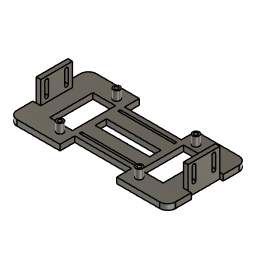
Plataforma_teorica_control_prueba v17 (Autodesk Fusion 360 design; units mm, degrees)
Autodesk Fusion 360 part; units mm, degrees
note: some values were not read from the file. Set by a fixed rule: which sketch regions a step uses.
sketch "Boceto1" plane through (0, 0, 0) normal (0, 0, 1) x (1, 0, 0)
  line L0 (0, 0) -> (80, 0) construction
  line L1 (80, 0) -> (80, 60) construction
  line L2 (80, 60) -> (0, 60) construction
  line L3 (0, 60) -> (0, 0) construction
  circle A0 centre (5, 55) radius 1.625
  circle A1 centre (75, 55) radius 1.625
  line L4 (110, -5) -> (-30, -5)
  line L5 (-30, -5) -> (-30, 65)
  line L6 (-30, 65) -> (110, 65)
  line L7 (110, 65) -> (110, -5)
  line L8 (15, 46) -> (65, 46)
  line L9 (65, 46) -> (65, 48)
  line L10 (65, 48) -> (15, 48)
  line L11 (15, 48) -> (15, 46)
  line L12 (-30, 30) -> (115, 30)
  line L13 (110, 30) -> (107, 30)
  line L14 (107, 30) -> (107, 44)
  line L15 (107, 44) -> (110, 44)
  line L16 (110, 44) -> (110, 30)
  line L17 (110, 16) -> (110, 30)
  line L18 (110, 30) -> (107, 30)
  line L19 (107, 16) -> (110, 16)
  line L20 (107, 30) -> (107, 16)
  line L21 (40, 65) -> (40, -5)
  circle A2 centre (5, 5) radius 1.625
  circle A3 centre (75, 5) radius 1.625
  line L22 (-30, 44) -> (-30, 30)
  line L23 (-30, 30) -> (-27, 30)
  line L24 (-27, 30) -> (-27, 44)
  line L25 (-27, 44) -> (-30, 44)
  line L26 (-30, 16) -> (-30, 30)
  line L27 (-30, 30) -> (-27, 30)
  line L28 (-27, 16) -> (-30, 16)
  line L29 (-27, 30) -> (-27, 16)
  line L30 (65, 12) -> (15, 12)
  line L31 (15, 12) -> (15, 14)
  line L32 (15, 14) -> (65, 14)
  line L33 (65, 14) -> (65, 12)
  dimension "d1" = 80
  dimension "d2" = 60
  dimension "d3" = 5
  dimension "d4" = 70
  dimension "d8" = 3.25
  dimension "d16" = 70
  dimension "d17" = 140
  dimension "d19" = 30
  dimension "d20" = 5
  dimension "d29" = 7
  dimension "d31" = 2
  dimension "d34" = 50
  dimension "d37" = 14
  dimension "d38" = 3
  dimension "d39" = 5
  constraint horizontal L0
  constraint vertical L1
  constraint horizontal L2
  constraint vertical L3
  constraint coincident L0.start L3.end
  constraint horizontal A0.centre A1.centre
  constraint equal A0 A1
  constraint horizontal L4
  constraint vertical L5
  constraint horizontal L6
  constraint vertical L7
  constraint horizontal L8
  constraint vertical L9
  constraint horizontal L10
  constraint vertical L11
  constraint midpoint L5 L12.start
  constraint horizontal L13
  constraint vertical L14
  constraint horizontal L15
  constraint vertical L16
  constraint midpoint L7 L13.start
  constraint symmetric L12 L13.start L16.end
  constraint symmetric L12 L13.end L14.start
  constraint symmetric L12 L14.end L19.start
  constraint symmetric L12 L15.end L17.start
  constraint perpendicular L5 L12
  constraint midpoint L6 L21.start
  constraint perpendicular L0 L21
  constraint midpoint L4 L21.end
  constraint symmetric A0 L12 A2
  constraint symmetric A1 L12 A3
  constraint symmetric L13.start L21 L12.start
  constraint symmetric L13.end L21 L23.end
  constraint symmetric L14.end L21 L24.end
  constraint symmetric L15.end L21 L22.start
  constraint symmetric L17.start L21 L26.start
  constraint symmetric L19.start L21 L28.start
  constraint symmetric L8.start L12 L31.end
  constraint symmetric L8.end L12 L32.end
  constraint symmetric L9.end L12 L30.start
  constraint symmetric L10.end L12 L30.end
  measures "d1" distance of L1.end L2.end
  measures "d2" distance of L0.end L1.end
  measures "d3" horizontal distance of L2.end A0.centre
  measures "d4" distance of A0.centre A1.centre
  measures "d8" diameter of A1
  measures "d16" distance of L4.start L6.end
  measures "d17" distance of L5.end L6.end
  measures "d19" horizontal distance of L0.end L4.start
  measures "d20" vertical distance of L0.end L4.start
  measures "d29" vertical distance of A0.centre L10.end
  measures "d31" distance of L8.end L9.end
  measures "d34" distance of L9.end L10.end
  measures "d37" distance of L13.start L15.end
  measures "d38" distance of L14.end L15.end
  measures "d39" vertical distance of L1.end A1.centre
extrude "Extruir1" add sketch "Boceto1" along normal blind 5 contours L4 L7 L12 L19 L20 L21 L30 L32 L33 | L4 L5 L12 L21 L28 L29 L30 L31 L32 | L6 L7 L8 L9 L10 L12 L14 L15 L21 | L5 L6 L8 L10 L11 L12 L21 L24 L25
sketch "Boceto4" plane through (0, 0, 5) normal (0, 0, 1) x (-1, 0, 0)
  line L0 (-15, -14) -> (-65, -14)
  line L1 (-65, -14) -> (-65, -12)
  line L2 (-65, -12) -> (-15, -12)
  line L3 (-15, -12) -> (-15, -14)
  circle A0 centre (-5, -5) radius 1.625
  circle A1 centre (-75, -55) radius 1.625
  circle A2 centre (-75, -5) radius 1.625
  circle A3 centre (-5, -55) radius 1.625
  line L4 (-15, -46) -> (-15, -48)
  line L5 (-15, -48) -> (-65, -48)
  line L6 (-65, -48) -> (-65, -46)
  line L7 (-65, -46) -> (-15, -46)
  line L8 (27, -44) -> (27, -16)
  line L9 (27, -16) -> (30, -16)
  line L10 (30, -16) -> (30, 5)
  line L11 (30, 5) -> (-110, 5)
  line L12 (-110, 5) -> (-110, -16)
  line L13 (-110, -16) -> (-107, -16)
  line L14 (-107, -16) -> (-107, -44)
  line L15 (-107, -44) -> (-110, -44)
  line L16 (-110, -44) -> (-110, -65)
  line L17 (-110, -65) -> (30, -65)
  line L18 (30, -65) -> (30, -44)
  line L19 (30, -44) -> (27, -44)
  line L20 (-107, -44) -> (-103, -44)
  line L21 (-103, -44) -> (-103, -16)
  line L22 (-103, -16) -> (-107, -16)
  line L23 (-107, -16) -> (-107, -44)
  line L24 (-40, -65) -> (-40, 5)
  line L25 (27, -30) -> (-107, -30)
  line L26 (27, -16) -> (27, -44)
  line L27 (27, -44) -> (23, -44)
  line L28 (23, -44) -> (23, -16)
  line L29 (23, -16) -> (27, -16)
  circle A4 centre (-5, -55) radius 3
  circle A5 centre (-75, -55) radius 3
  circle A6 centre (-5, -5) radius 3
  circle A7 centre (-75, -5) radius 3
  dimension "d42" = 4
  dimension "d58" = 6
  constraint horizontal L20
  constraint vertical L21
  constraint horizontal L22
  constraint vertical L23
  constraint coincident L14.end L15.start
  constraint midpoint L17 L24.start
  constraint midpoint L11 L24.end
  constraint midpoint L8 L25.start
  constraint coincident L13.end L14.start
  constraint symmetric L14.end L24 L8.start
  constraint symmetric L20.end L24 L27.end
  constraint symmetric L21.end L24 L28.end
  constraint symmetric L13.end L24 L8.end
  constraint horizontal L25
  constraint midpoint L23 L25.end
  constraint concentric A3 A4
  constraint symmetric L24 A4 A5
  constraint symmetric L25 A4 A6
  constraint symmetric L25 A5 A7
  measures "d42" distance of L14.end L20.end
  measures "d58" diameter of A4
extrude "Extruir3" add sketch "Boceto4" along normal blind 20 contours L8 L25 L26 L28 L29 | L8 L25 L26 L27 L28 | L14 L21 L22 L23 L25 | L14 L20 L21 L23 L25
extrude "Extruir2" add sketch "Boceto4" along normal blind 10 contours L8 L25 L26 L28 L29 | L8 L25 L26 L27 L28 | L14 L21 L22 L23 L25 | L14 L20 L21 L23 L25
sketch "Boceto5" plane through (107, 0, 0) normal (1, 0, 0) x (0, 1, 0)
  line L0 (16, 0) -> (44, 0)
  line L1 (44, 0) -> (44, 5)
  line L2 (44, 5) -> (44, 25)
  line L3 (16, 25) -> (16, 5)
  line L4 (16, 5) -> (16, 0)
  line L5 (30, 25) -> (30, 0)
  line L6 (44, 25) -> (16, 25)
  line L7 (19.65, 21.5) -> (19.65, 9.5)
  arc A0 (19.65, 9.5) -> (22.85, 9.5) centre (21.25, 9.5) ccw
  line L8 (22.85, 9.5) -> (22.85, 21.5)
  arc A1 (22.85, 21.5) -> (19.65, 21.5) centre (21.25, 21.5) ccw
  line L9 (21.25, 21.5) -> (21.25, 9.5) construction
  arc A2 (37.15, 9.5) -> (40.35, 9.5) centre (38.75, 9.5) ccw
  line L10 (37.15, 9.5) -> (37.15, 21.5)
  arc A3 (40.35, 21.5) -> (37.15, 21.5) centre (38.75, 21.5) ccw
  line L11 (40.35, 21.5) -> (40.35, 9.5)
  dimension "d52" = 3.2
  dimension "d53" = 12
  dimension "d54" = 8.75
  dimension "d55" = 3.5
  constraint midpoint L5.start L6
  constraint midpoint L0 L5.end
  constraint tangent L7 A0
  constraint tangent A0 L8
  constraint parallel L7 L8
  constraint tangent L8 A1
  constraint tangent L7 A1
  constraint vertical L9
  constraint symmetric L5 L7.start A3.start
  constraint symmetric L5 L7.end A2.end
  constraint symmetric L5 A0.end A2.start
  constraint symmetric L5 L8.end L10.end
  constraint symmetric L5 A0 A2
  constraint symmetric L5 A1 A3
  measures "d52" diameter of A0
  measures "d53" distance of A1.centre A0.centre
  measures "d54" horizontal distance of L5.start A1.centre
  measures "d55" vertical distance of L5.start A1.centre
sketch "Boceto2" plane through (0, 0, 0) normal (0, 0, 1) x (1, 0, 0)
sketch "Boceto3" plane through (0, 0, 0) normal (0, 0, 1) x (1, 0, 0)
  point P0 (5, 55)
extrude "Extruir4" cut sketch "Boceto5" against normal blind 155 contours L7 A0 L8 A1 | A2 L10 A3 L11
extrude "Extruir5" add sketch "Boceto4" along normal blind 8 contours A4 | A5 | A6 | A7
sketch "Boceto6" plane through (0, 0, 5) normal (0, 0, 1) x (-1, 0, 0)
  line L0 (10, -30) -> (-10, -30)
  line L1 (-10, -30) -> (-10, -49)
  line L2 (-10, -49) -> (10, -49)
  line L3 (10, -49) -> (10, -30)
  line L4 (-15, -65) -> (-40, -65)
  line L5 (-40, -65) -> (-40, -52)
  line L6 (-40, -52) -> (-15, -52)
  line L7 (-15, -52) -> (-15, -65)
  line L8 (-40, -65) -> (-40, 5)
  line L9 (-90, -49) -> (-90, -30)
  line L10 (-90, -30) -> (-70, -30)
  line L11 (-70, -30) -> (-70, -49)
  line L12 (-70, -49) -> (-90, -49)
  line L13 (27, -30) -> (-107, -30)
  line L14 (-10, -30) -> (-10, -11)
  line L15 (-10, -11) -> (10, -11)
  line L16 (10, -11) -> (10, -30)
  line L17 (10, -30) -> (-10, -30)
  line L18 (-70, -30) -> (-70, -11)
  line L19 (-70, -11) -> (-90, -11)
  line L20 (-90, -11) -> (-90, -30)
  line L21 (-90, -30) -> (-70, -30)
  line L22 (-65, -65) -> (-40, -65)
  line L23 (-40, -65) -> (-40, -52)
  line L24 (-40, -52) -> (-65, -52)
  line L25 (-65, -52) -> (-65, -65)
  line L26 (-15, 5) -> (-40, 5)
  line L27 (-40, 5) -> (-40, -8)
  line L28 (-40, -8) -> (-15, -8)
  line L29 (-15, -8) -> (-15, 5)
  line L30 (-40, -8) -> (-65, -8)
  line L31 (-65, -8) -> (-65, 5)
  line L32 (-65, 5) -> (-40, 5)
  line L33 (-40, 5) -> (-40, -8)
  line L34 (-40, -30) -> (-16, -30)
  line L35 (-16, -30) -> (-16, -35)
  line L36 (-16, -35) -> (-40, -35)
  line L37 (-40, -35) -> (-40, -30)
  line L38 (-40, -30) -> (-64, -30)
  line L39 (-64, -30) -> (-64, -35)
  line L40 (-40, -35) -> (-40, -30)
  line L41 (-64, -35) -> (-40, -35)
  line L42 (-40, -30) -> (-16, -30)
  line L43 (-16, -30) -> (-16, -25)
  line L44 (-16, -25) -> (-40, -25)
  line L45 (-40, -25) -> (-40, -30)
  line L46 (-40, -30) -> (-64, -30)
  line L47 (-64, -30) -> (-64, -25)
  line L48 (-64, -25) -> (-40, -25)
  line L49 (-40, -25) -> (-40, -30)
  arc A0 (-103, 5) -> (-110, -2) centre (-103, -2) ccw
  line L50 (-103, 5) -> (-110, 5)
  line L51 (-110, 5) -> (-110, -2)
  line L52 (30, 5) -> (30, -2)
  line L53 (23, 5) -> (30, 5)
  arc A1 (30, -2) -> (23, 5) centre (23, -2) ccw
  line L54 (-110, -65) -> (-110, -58)
  line L55 (-103, -65) -> (-110, -65)
  arc A2 (-110, -58) -> (-103, -65) centre (-103, -58) ccw
  line L56 (30, -65) -> (30, -58)
  arc A3 (23, -65) -> (30, -58) centre (23, -58) ccw
  line L57 (23, -65) -> (30, -65)
  point P0 (-5, -55)
  point P1 (-75, -5)
  point P2 (-110, 5)
  dimension "d61" = 15
  dimension "d62" = 6
  dimension "d63" = 19
  dimension "d64" = 20
  dimension "d65" = 25
  dimension "d66" = 13
  dimension "d67" = 24
  dimension "d68" = 5
  dimension "d72" = 7
  dimension "d73" = 3
  constraint horizontal L0
  constraint vertical L1
  constraint horizontal L2
  constraint vertical L3
  constraint horizontal L4
  constraint vertical L5
  constraint horizontal L6
  constraint vertical L7
  constraint symmetric L0.start L8 L9.end
  constraint symmetric L0.end L8 L10.end
  constraint symmetric L1.end L8 L11.end
  constraint symmetric L2.end L8 L9.start
  constraint symmetric L0.start L13 L3.end
  constraint symmetric L0.end L13 L1.start
  constraint symmetric L1.end L13 L14.end
  constraint symmetric L2.end L13 L15.end
  constraint symmetric L9.start L13 L19.end
  constraint symmetric L9.end L13 L10.start
  constraint symmetric L10.end L13 L11.start
  constraint symmetric L11.end L13 L18.end
  constraint coincident L4.end L5.start
  constraint symmetric L4.start L8 L22.start
  constraint symmetric L4.end L8 L5.start
  constraint symmetric L5.end L8 L6.start
  constraint symmetric L6.end L8 L24.end
  constraint symmetric L4.start L13 L26.start
  constraint symmetric L4.end L13 L8.end
  constraint symmetric L5.end L13 L27.end
  constraint symmetric L6.end L13 L28.end
  constraint symmetric L13 L22.start L31.end
  constraint symmetric L13 L4.end L8.end
  constraint symmetric L13 L5.end L27.end
  constraint symmetric L13 L24.end L30.end
  constraint horizontal L34
  constraint vertical L35
  constraint horizontal L36
  constraint vertical L37
  constraint midpoint L13 L34.start
  constraint symmetric L8 L34.start L37.end
  constraint symmetric L8 L34.end L38.end
  constraint symmetric L8 L35.end L39.end
  constraint symmetric L8 L36.end L37.start
  constraint symmetric L13 L34.start L37.end
  constraint symmetric L13 L34.end L35.start
  constraint symmetric L13 L35.end L43.end
  constraint symmetric L13 L36.end L44.end
  constraint symmetric L13 L38.end L39.start
  constraint symmetric L13 L39.end L47.end
  constraint tangent A0 L50
  constraint horizontal L50
  constraint tangent A0 L51
  constraint horizontal A0.centre A0.end
  constraint symmetric L8 A0.start L53.start
  constraint symmetric L8 A0.end L52.end
  constraint symmetric L8 A0 A1
  constraint symmetric L8 P2 L52.start
  constraint symmetric L13 A0.start L55.start
  constraint symmetric L13 A0.end L54.end
  constraint symmetric L13 A0 A2
  constraint symmetric L13 P2 L54.start
  constraint symmetric L8 L54.start L56.start
  constraint symmetric L8 L54.end L56.end
  constraint symmetric L8 L55.start A3.start
  constraint symmetric L8 A2 A3
  constraint coincident P2 L50.end
  measures "d61" horizontal distance of L2.end P0
  measures "d62" vertical distance of L1.end P0
  measures "d63" distance of L0.end L1.end
  measures "d64" distance of L1.end L2.end
  measures "d65" distance of L4.start L4.end
  measures "d66" distance of L4.start L6.end
  measures "d67" distance of L35.end L36.end
  measures "d68" distance of L34.end L35.end
  measures "d72" distance of A0.centre A0.start
  measures "d73" vertical distance of A0.centre P1
extrude "Extruir6" cut sketch "Boceto6" against normal blind 25 contours L0 L1 L2 L3 L13 L17 | L0 L13 L14 L15 L16 L17 | L4 L5 L6 L7 L8 L23 | L5 L8 L22 L23 L24 L25 | L8 L13 L37 L38 L39 L40 L41 L46 | L8 L13 L34 L35 L36 L37 L40 L42 | L8 L13 L38 L45 L46 L47 L48 L49 | L8 L13 L34 L42 L43 L44 L45 L49 | L8 L27 L30 L31 L32 L33 | L8 L26 L27 L28 L29 L33 | L9 L10 L11 L12 L13 L21 | L10 L13 L18 L19 L20 L21
extrude "Extruir7" cut sketch "Boceto6" against normal blind 15 contours A0 L50 L51 | L52 L53 A1 | L54 L55 A2 | L56 A3 L57
equation "d37 = ( 28 / 2 ) * 1 mm"
equation "d54 = ( 17.5 / 2 ) * 1 mm"
